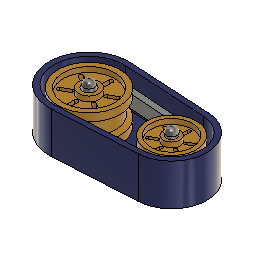
PULLEY LEZIONE v5 (Autodesk Fusion 360 design; units mm, degrees)
Autodesk Fusion 360 part; units mm, degrees
sketch "Schizzo1" plane through (0, 0, 0) normal (0, 1, 0) x (1, 0, 0) in component "PULEGGIA GRANDE"
  line L0 (-10.2679, 0) -> (-10.2679, -2.5)
  line L1 (-10.2679, -2.5) -> (-12, -3.5)
  line L2 (-12, -3.5) -> (-12, -6.5)
  line L3 (-12, -6.5) -> (0, -6.5)
  line L4 (0, -6.5) -> (0, 0)
  line L5 (-10.2679, 0) -> (0, 0) construction
  line L6 (-10.2679, 0) -> (-10.2679, 2.5)
  line L7 (-10.2679, 2.5) -> (-12, 3.5)
  line L8 (-12, 3.5) -> (-12, 6.5)
  line L9 (-12, 6.5) -> (0, 6.5)
  line L10 (0, 6.5) -> (0, 0)
  dimension "d1" = 2.5
  dimension "d2" = 3
  dimension "d3" = 2
  dimension "d4" = 12
  constraint vertical L0
  constraint parallel L0 L2
  constraint perpendicular L0 L3
  constraint coincident L4.end L5.end
  constraint perpendicular L3 L4
  constraint perpendicular L4 L5
  constraint symmetric L0.start L5 L6.start
  constraint symmetric L0.end L5 L6.end
  constraint symmetric L1.end L5 L7.end
  constraint symmetric L2.end L5 L8.end
  constraint symmetric L3.end L5 L9.end
  constraint symmetric L4.end L5 L10.end
  measures "d1" distance of L0.start L0.end
  measures "d2" distance of L1.end L2.end
  measures "d3" distance of L0.end L1.end
  measures "d4" distance of L2.end L3.end
revolve "Rivoluzione1" add sketch "Schizzo1" angle 360 about axis through (0, 0, 6.5) along (0, 0, -1) makes body 1 in component "PULEGGIA GRANDE"
sketch "Schizzo2" plane through (0, 0, 6.5) normal (0, 0, 1) x (-1, 0, 0) in component "PULEGGIA GRANDE"
  circle A0 centre (0, 0) radius 12
  circle A1 centre (0, 0) radius 10
  circle A2 centre (0, 0) radius 4
  circle A3 centre (0, 0) radius 2.5
  line L0 (0.7882, -8.551) -> (0.7882, -5)
  arc A4 (0.7882, -5) -> (-0.7118, -5) centre (0.0382, -5) ccw
  line L1 (-0.7118, -5) -> (-0.7118, -8.551)
  arc A5 (-0.7118, -8.551) -> (0.7882, -8.551) centre (0.0382, -8.551) ccw
  line L2 (0.0382, -8.551) -> (0.0382, -5) construction
  dimension "d6" = 20
  dimension "d7" = 8
  dimension "d8" = 5
  dimension "d9" = 1.5
  constraint coincident A0.centre A1.centre
  constraint tangent L0 A4
  constraint tangent A4 L1
  constraint parallel L0 L1
  constraint tangent L1 A5
  constraint tangent L0 A5
  constraint vertical L2
  measures "d6" diameter of A1
  measures "d7" diameter of A2
  measures "d8" diameter of A3
  measures "d9" diameter of A4
extrude "Estrudi1" cut sketch "Schizzo2" against normal blind 2 contours A1 bodies 1 in component "PULEGGIA GRANDE"
extrude "Estrudi2" cut sketch "Schizzo2" against normal blind 23 contours A3 bodies 1 in component "PULEGGIA GRANDE"
extrude "Estrudi3" cut sketch "Schizzo2" against normal blind 26 contours L0 A4 L1 A5 bodies 1 in component "PULEGGIA GRANDE"
pattern_circular "Serie C1" count 6 over 360 about axis through (0, 0, 6.5) along (0, 0, 1) of "Estrudi3" in component "PULEGGIA GRANDE"
sketch "Schizzo1 (2)" plane through (0, 0, 0) normal (0, 1, 0) x (1, 0, 0) in component "PULEGGIA PICCOLA"
  line L0 (-10.2679, 0) -> (-10.2679, -2.5)
  line L1 (-10.2679, -2.5) -> (-12, -3.5)
  line L2 (-12, -3.5) -> (-12, -6.5)
  line L3 (-12, -6.5) -> (0, -6.5)
  line L4 (0, -6.5) -> (0, 0)
  line L5 (-10.2679, 0) -> (0, 0) construction
  line L6 (-10.2679, 0) -> (-10.2679, 2.5)
  line L7 (-10.2679, 2.5) -> (-12, 3.5)
  line L8 (-12, 3.5) -> (-12, 6.5)
  line L9 (-12, 6.5) -> (0, 6.5)
  line L10 (0, 6.5) -> (0, 0)
  dimension "d1_1" = 2.5
  dimension "d2_1" = 3
  dimension "d3_1" = 2
  dimension "d4_1" = 12
  constraint vertical L0
  constraint parallel L0 L2
  constraint perpendicular L0 L3
  constraint coincident L4.end L5.end
  constraint perpendicular L3 L4
  constraint perpendicular L4 L5
  constraint symmetric L0.start L5 L6.start
  constraint symmetric L0.end L5 L6.end
  constraint symmetric L1.end L5 L7.end
  constraint symmetric L2.end L5 L8.end
  constraint symmetric L3.end L5 L9.end
  constraint symmetric L4.end L5 L10.end
  measures "d1_1" distance of L0.start L0.end
  measures "d2_1" distance of L1.end L2.end
  measures "d3_1" distance of L0.end L1.end
  measures "d4_1" distance of L2.end L3.end
revolve "Rivoluzione1'" add sketch "Schizzo1 (2)" angle 360 about axis through (0, 0, 6.5) along (0, 0, -1) separate body makes body 2 in component "PULEGGIA PICCOLA"
sketch "Schizzo2 (2)" plane through (0, 0, 6.5) normal (0, 0, 1) x (-1, 0, 0) in component "PULEGGIA PICCOLA"
  circle A0 centre (0, 0) radius 12
  circle A1 centre (0, 0) radius 10
  circle A2 centre (0, 0) radius 4
  circle A3 centre (0, 0) radius 2.5
  line L0 (0.7882, -8.551) -> (0.7882, -5)
  arc A4 (0.7882, -5) -> (-0.7118, -5) centre (0.0382, -5) ccw
  line L1 (-0.7118, -5) -> (-0.7118, -8.551)
  arc A5 (-0.7118, -8.551) -> (0.7882, -8.551) centre (0.0382, -8.551) ccw
  line L2 (0.0382, -8.551) -> (0.0382, -5) construction
  dimension "d6_1" = 20
  dimension "d7_1" = 8
  dimension "d8_1" = 5
  dimension "d9_1" = 1.5
  constraint coincident A0.centre A1.centre
  constraint tangent L0 A4
  constraint tangent A4 L1
  constraint parallel L0 L1
  constraint tangent L1 A5
  constraint tangent L0 A5
  constraint vertical L2
  measures "d6_1" diameter of A1
  measures "d7_1" diameter of A2
  measures "d8_1" diameter of A3
  measures "d9_1" diameter of A4
extrude "Estrudi1'" cut sketch "Schizzo2 (2)" against normal blind 2 contours A1 bodies 2 in component "PULEGGIA PICCOLA"
extrude "Estrudi2'" cut sketch "Schizzo2 (2)" against normal blind 23 contours A3 bodies 2 in component "PULEGGIA PICCOLA"
extrude "Estrudi3'" cut sketch "Schizzo2 (2)" against normal blind 26 contours L0 A4 L1 A5 bodies 2 in component "PULEGGIA PICCOLA"
pattern_circular "Serie C1'" count 6 over 360 about axis through (0, 0, 6.5) along (0, 0, 1) of "Estrudi3'" in component "PULEGGIA PICCOLA"
scale "Scala1" factors (0.8, 0.8, 1) about (10, 0, 4.5) bodies 2 in component "PULEGGIA PICCOLA"
sketch "Schizzo1 (3)" plane through (0, 0, 6.5) normal (0, 0, 1) x (-1, 0, 0)
  circle A0 centre (0, 0) radius 10
  circle A1 centre (0, 0) radius 12
  line L0 (-4.686, -1.8835) -> (-7.7613, -3.6591)
  arc A2 (-3.936, -3.1826) -> (-4.686, -1.8835) centre (-4.311, -2.5331) ccw
  line L1 (-7.0113, -4.9581) -> (-3.936, -3.1826)
  arc A3 (-7.7613, -3.6591) -> (-7.0113, -4.9581) centre (-7.3863, -4.3086) ccw
  line L2 (-3.9742, 3.1165) -> (-7.0495, 4.892)
  arc A4 (-4.7242, 1.8174) -> (-3.9742, 3.1165) centre (-4.3492, 2.4669) ccw
  line L3 (-7.7995, 3.5929) -> (-4.7242, 1.8174)
  arc A5 (-7.0495, 4.892) -> (-7.7995, 3.5929) centre (-7.4245, 4.2424) ccw
  line L4 (0.7118, 5) -> (0.7118, 8.551)
  arc A6 (-0.7882, 5) -> (0.7118, 5) centre (-0.0382, 5) ccw
  line L5 (-0.7882, 8.551) -> (-0.7882, 5)
  arc A7 (0.7118, 8.551) -> (-0.7882, 8.551) centre (-0.0382, 8.551) ccw
  line L6 (4.686, 1.8835) -> (7.7613, 3.6591)
  arc A8 (3.936, 3.1826) -> (4.686, 1.8835) centre (4.311, 2.5331) ccw
  line L7 (7.0113, 4.9581) -> (3.936, 3.1826)
  arc A9 (7.7613, 3.6591) -> (7.0113, 4.9581) centre (7.3863, 4.3086) ccw
  line L8 (3.9742, -3.1165) -> (7.0495, -4.892)
  arc A10 (4.7242, -1.8174) -> (3.9742, -3.1165) centre (4.3492, -2.4669) ccw
  line L9 (7.7995, -3.5929) -> (4.7242, -1.8174)
  arc A11 (7.0495, -4.892) -> (7.7995, -3.5929) centre (7.4245, -4.2424) ccw
  line L10 (-0.7118, -5) -> (-0.7118, -8.551)
  arc A12 (-0.7118, -8.551) -> (0.7882, -8.551) centre (0.0382, -8.551) ccw
  line L11 (0.7882, -8.551) -> (0.7882, -5)
  arc A13 (0.7882, -5) -> (-0.7118, -5) centre (0.0382, -5) ccw
  circle A14 centre (0, 0) radius 2.5
  circle A15 centre (0, 0) radius 12
  line L12 (-35.7488, -1.5068) -> (-38.209, -2.9272)
  arc A16 (-35.1488, -2.5461) -> (-35.7488, -1.5068) centre (-35.4488, -2.0265) ccw
  line L13 (-37.609, -3.9665) -> (-35.1488, -2.5461)
  arc A17 (-38.209, -2.9272) -> (-37.609, -3.9665) centre (-37.909, -3.4469) ccw
  line L14 (-35.1794, 2.4932) -> (-37.6396, 3.9136)
  arc A18 (-35.7794, 1.4539) -> (-35.1794, 2.4932) centre (-35.4794, 1.9735) ccw
  line L15 (-38.2396, 2.8743) -> (-35.7794, 1.4539)
  arc A19 (-37.6396, 3.9136) -> (-38.2396, 2.8743) centre (-37.9396, 3.394) ccw
  line L16 (-31.4305, 4) -> (-31.4305, 6.8408)
  arc A20 (-32.6305, 4) -> (-31.4305, 4) centre (-32.0305, 4) ccw
  line L17 (-32.6305, 6.8408) -> (-32.6305, 4)
  arc A21 (-31.4305, 6.8408) -> (-32.6305, 6.8408) centre (-32.0305, 6.8408) ccw
  line L18 (-28.2512, 1.5068) -> (-25.791, 2.9272)
  arc A22 (-28.8512, 2.5461) -> (-28.2512, 1.5068) centre (-28.5512, 2.0265) ccw
  line L19 (-26.391, 3.9665) -> (-28.8512, 2.5461)
  arc A23 (-25.791, 2.9272) -> (-26.391, 3.9665) centre (-26.091, 3.4469) ccw
  line L20 (-28.8206, -2.4932) -> (-26.3604, -3.9136)
  arc A24 (-28.2206, -1.4539) -> (-28.8206, -2.4932) centre (-28.5206, -1.9735) ccw
  line L21 (-25.7604, -2.8743) -> (-28.2206, -1.4539)
  arc A25 (-26.3604, -3.9136) -> (-25.7604, -2.8743) centre (-26.0604, -3.394) ccw
  line L22 (-32.5695, -4) -> (-32.5695, -6.8408)
  arc A26 (-32.5695, -6.8408) -> (-31.3695, -6.8408) centre (-31.9695, -6.8408) ccw
  line L23 (-31.3695, -6.8408) -> (-31.3695, -4)
  arc A27 (-31.3695, -4) -> (-32.5695, -4) centre (-31.9695, -4) ccw
  circle A28 centre (-32, 0) radius 2
  circle A29 centre (-32, 0) radius 9.6
  line L24 (-0.915, -12.1656) -> (-32.735, -9.7724)
  line L25 (-0.915, 12.1656) -> (-32.735, 9.7724)
  arc A30 (-0.915, -12.1656) -> (-0.915, 12.1656) centre (0, 0) ccw
  arc A31 (-32.735, 9.7724) -> (-32.735, -9.7724) centre (-32, 0) ccw
  constraint tangent L24 A30
  constraint tangent L24 A31
  constraint tangent L25 A31
  constraint tangent L25 A30
  constraint concentric A1 A30
  constraint concentric A29 A31
sketch "Schizzo2 (3)" plane through (0, 0, 0) normal (0, 1, 0) x (1, 0, 0)
  line L0 (-12, -2.866) -> (-10.5, -2)
  line L1 (-10.5, -2) -> (-10.5, 3)
  line L2 (-10.5, 3) -> (-12, 3.866)
  line L3 (-12, 3.866) -> (-12, -2.866)
  dimension "d23" = 120
  dimension "d24" = 120
  dimension "d25" = 5
  constraint vertical L1
  constraint parallel L1 L3
  measures "d23" angle of L0 L1
  measures "d24" angle of L1 L2
  measures "d25" distance of L0.end L1.end
sweep "Sweep1" add profiles "Schizzo2 (3)" path "Schizzo1 (3)" along A31 L24 A30 L25 section 1 separate body makes body 3
move_body "Sposta1" bodies 3 to x (1, 0, 0) y (0, 1, 0) z (0, 0, 1) at (0, 0, 0.5)
sketch "Schizzo3" plane through (0, 0, -6.5) normal (0, 0, -1) x (1, 0, 0)
  line L0 (7.0113, -4.9581) -> (3.936, -3.1826)
  arc A0 (4.686, -1.8835) -> (3.936, -3.1826) centre (4.311, -2.5331) ccw
  line L1 (4.686, -1.8835) -> (7.7613, -3.6591)
  arc A1 (7.0113, -4.9581) -> (7.7613, -3.6591) centre (7.3863, -4.3086) ccw
  line L2 (7.7995, 3.5929) -> (4.7242, 1.8174)
  arc A2 (3.9742, 3.1165) -> (4.7242, 1.8174) centre (4.3492, 2.4669) ccw
  line L3 (3.9742, 3.1165) -> (7.0495, 4.892)
  arc A3 (7.7995, 3.5929) -> (7.0495, 4.892) centre (7.4245, 4.2424) ccw
  line L4 (0.7882, 8.551) -> (0.7882, 5)
  arc A4 (-0.7118, 5) -> (0.7882, 5) centre (0.0382, 5) ccw
  line L5 (-0.7118, 5) -> (-0.7118, 8.551)
  arc A5 (0.7882, 8.551) -> (-0.7118, 8.551) centre (0.0382, 8.551) ccw
  line L6 (-7.0113, 4.9581) -> (-3.936, 3.1826)
  arc A6 (-4.686, 1.8835) -> (-3.936, 3.1826) centre (-4.311, 2.5331) ccw
  line L7 (-4.686, 1.8835) -> (-7.7613, 3.6591)
  arc A7 (-7.0113, 4.9581) -> (-7.7613, 3.6591) centre (-7.3863, 4.3086) ccw
  line L8 (-7.7995, -3.5929) -> (-4.7242, -1.8174)
  arc A8 (-3.9742, -3.1165) -> (-4.7242, -1.8174) centre (-4.3492, -2.4669) ccw
  line L9 (-3.9742, -3.1165) -> (-7.0495, -4.892)
  arc A9 (-7.7995, -3.5929) -> (-7.0495, -4.892) centre (-7.4245, -4.2424) ccw
  line L10 (-0.7882, -8.551) -> (-0.7882, -5)
  arc A10 (0.7118, -5) -> (-0.7882, -5) centre (-0.0382, -5) ccw
  line L11 (0.7118, -5) -> (0.7118, -8.551)
  arc A11 (-0.7882, -8.551) -> (0.7118, -8.551) centre (-0.0382, -8.551) ccw
  circle A12 centre (0, 0) radius 2.5
  circle A13 centre (0, 0) radius 12
  circle A14 centre (0, 0) radius 14
  circle A15 centre (32, 0) radius 11
  line L12 (-0.1538, 13.9992) -> (32, 11)
  line L13 (0.0009, -14) -> (32, -11)
  dimension "d32" = 28
  dimension "d33" = 22
  constraint concentric A12 A14
  constraint coincident A14 L12.start
  constraint coincident A15 L12.end
  constraint coincident A14 L13.start
  constraint coincident A15 L13.end
  measures "d32" diameter of A14
  measures "d33" diameter of A15
ref_plane "Piano di lavoro1" through (0, 0, -6.5) normal (0, 0, -1) x (-1, 0, 0)
sketch "Schizzo4" plane through (0, 0, -6.5) normal (0, 0, -1) x (1, 0, 0)
  line L0 (0.7533, -13.4325) -> (32.653, -11.6436)
  line L1 (0.7533, 13.4325) -> (32.653, 11.6436)
  arc A0 (0.7533, 13.4325) -> (0.7533, -13.4325) centre (0, 0) ccw
  arc A1 (32.653, -11.6436) -> (32.653, 11.6436) centre (32, 0) ccw
  constraint coincident A0.centre origin
  constraint tangent L0 A0
  constraint tangent L1 A0
  constraint tangent L1 A1
  constraint tangent L0 A1
extrude "Estrudi1''" add sketch "Schizzo4" against normal blind 14 separate body makes body 4
shell "Shell1" thickness 2 outward yes removed faces 1 at (11.3865, -3.8812, 7.5) on bodies 4
sketch "Schizzo5" plane through (0, 0, -6.5) normal (0, 0, 1) x (-1, 0, 0)
  arc A0 (-0.7533, -13.4325) -> (-0.7533, 13.4325) centre (0, 0) ccw
  line L0 (-0.7533, 13.4325) -> (-32.653, 11.6436)
  arc A1 (-32.653, 11.6436) -> (-32.653, -11.6436) centre (-32, 0) ccw
  line L1 (-32.653, -11.6436) -> (-0.7533, -13.4325)
  circle A2 centre (0, 0) radius 2.1
  circle A3 centre (-32, 0) radius 2.1
  dimension "d38" = 4.2
  dimension "d39" = 4.2
  constraint coincident A0.centre A2.centre
  constraint concentric A1 A3
  measures "d38" diameter of A2
  measures "d39" diameter of A3
extrude "Estrudi2''" add sketch "Schizzo5" along normal blind 16 separate body contours A2 | A3 makes body 5 at (-2.0974, 0.1047, 4.1667) makes body 6 at (29.9026, 0.1047, 4.1667)
fillet "Raccordo1" radius 2 2 edges at (1.9579, 0.7594, 9.5) (33.9579, 0.7594, 9.5) on bodies 5 6
copy_body "Corpo->Comp1" bodies 4 removing the originals makes body 7 in component "BASE"
component "PULEGGIA GRANDE" placed x (0.999974, -0.007257, 0) y (0.007257, 0.999974, 0) z (0, 0, 1) at (0, 0, 0)
component "PULEGGIA PICCOLA" placed x (0.999998, 0.002137, 0) y (-0.002137, 0.999998, 0) z (0, 0, 1) at (30, -0.0045, 0)
component "BASE" placed x (1, 0, 0) y (0, 1, 0) z (0, 0, 1) at (0, 0, 0)
